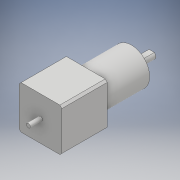
# Autodesk Inventor part: Base_Motor
Saved by Autodesk Inventor 2018 (Build 220112000, 112)
## iProperties
Created: 2018-11-04
Part Number: Base_Motor
Material: Generic
Document SubType Name: Modeling
Designer: Cameron
Density: 1 g/cm^3
Appearance: Default
Author: Cameron
Autodesk Inventor part; units mm, degrees
ref_plane "YZ Plane" through (0, 0, 0) normal (1, 0, 0) x (0, 1, 0)
ref_plane "XZ Plane" through (0, 0, 0) normal (0, 1, 0) x (-1, 0, 0)
ref_plane "XY Plane" through (0, 0, 0) normal (0, 0, 1) x (1, 0, 0)
sketch "Sketch1" plane through (0, 0, 0) normal (1, 0, 0) x (0, 1, 0)
  line L0 (22.9102, 23.0555) -> (-21.7898, 23.0555)
  line L1 (-21.7898, 23.0555) -> (-21.7898, -19.2445)
  line L2 (-21.7898, -19.2445) -> (22.9102, -19.2445)
  line L3 (22.9102, -19.2445) -> (22.9102, 23.0555)
  point P0 (0, 0)
  dimension "d0" = 44.7
  dimension "d1" = 42.3
  constraints: 8 end point, 2 parallel, 1 horizontal, 1 perpendicular
  measures "d0" distance of L1.end L2.end
  measures "d1" distance of L2.end L0.start
extrude "Extrusion1" add sketch "Sketch1" along normal blind 42.3
sketch "Sketch2" plane through (0, 22.9102, 23.0555) normal (0, 1, 0) x (1, 0, 0)
  line L0 (0, 42.3) -> (0, 0) projected
  line L1 (0, 0) -> (42.3, 0) projected
  line L2 (42.3, 42.3) -> (42.3, 0) projected
  line L3 (0, 42.3) -> (42.3, 42.3) projected
  circle A0 centre (21.15, 21.15) radius 18
  point P0 (0, 23.0555)
  dimension "d4" = 21.15
  dimension "d5" = 36
  constraints: 1 centre point
  measures "d4" distance from line of L3 A0.centre
  measures "d5" diameter of A0
extrude "Extrusion2" add sketch "Sketch2" along normal blind 45 contours A0
sketch "Sketch3" plane through (21.15, 67.9102, 1.9055) normal (0, 1, 0) x (1, 0, 0)
  circle A0 centre (0, 0) radius 18 projected
  circle A1 centre (0, 0) radius 11
  point P0 (-21.15, 1.9055)
  dimension "d8" = 22
  constraints: 1 centre point, 1 coincident
  measures "d8" diameter of A1
extrude "Extrusion3" add sketch "Sketch3" along normal blind 2 contours A1
sketch "Sketch4" plane through (21.15, 69.9102, 1.9055) normal (0, 1, 0) x (1, 0, 0)
  circle A0 centre (0, 0) radius 11 projected
  circle A1 centre (0, 0) radius 4
  point P0 (-21.15, 1.9055)
  dimension "d11" = 8
  constraints: 1 centre point, 1 coincident
  measures "d11" diameter of A1
extrude "Extrusion4" add sketch "Sketch4" along normal blind 3 contours A1
sketch "Sketch5" plane through (21.15, 72.9102, 1.9055) normal (0, 1, 0) x (1, 0, 0)
  circle A0 centre (0, 0) radius 4 projected
  circle A1 centre (0, 0) radius 4
  line L0 (-2.6458, -3) -> (2.6458, -3)
  circle A2 centre (0, 0) radius 4 projected
  line L1 (-21.15, -21.15) -> (21.15, -21.15) projected
  line L2 (0, -4) -> (21.15, -4)
  line L3 (21.15, 21.15) -> (21.15, -21.15) projected
  point P0 (-21.15, 1.9055)
  dimension "d14" = 1
  dimension "d15" = 1
  constraints: 4 end point, 2 point on circle, 1 coincident, 1 horizontal, 1 point on line, 4 other
  measures "d14" vertical distance of L0.start L2.start
  measures "d15" vertical distance of L0.end L2.end
extrude "Extrusion5" add sketch "Sketch5" along normal blind 15 contours A0 L0 picked at (1.0912, -0.393)
sketch "Sketch6" plane through (0, -21.7898, -19.2445) normal (0, -1, 0) x (1, 0, 0)
  circle A0 centre (21.15, 21.15) radius 4 projected
  circle A1 centre (21.15, 21.15) radius 1.95
  point P0 (0, 19.2445)
  dimension "d18" = 3.9
  constraints: 1 centre point, 1 coincident
  measures "d18" diameter of A1
extrude "Extrusion6" add sketch "Sketch6" along normal blind 12 contours A1
chamfer "Chamfer1" distance 2 angle 45 4 edges at (42.3, 0.5602, 23.0555) (0, 0.5602, 23.0555) (42.3, 0.5602, -19.2445) (0, 0.5602, -19.2445)
body "Solid1"
